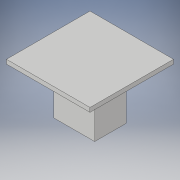
# Autodesk Inventor part: Beacon-Support
Saved by Autodesk Inventor 2017.3 (Build 213256000, 256)
## iProperties
Part Number: Beacon-Support
Material: Generisch
Document SubType Name: Modeling
Designer: Nils
Density: 1 g/cm^3
Appearance: Vorgabe
Author: Nils
Autodesk Inventor part; units mm, degrees
ref_plane "YZ Plane" through (0, 0, 0) normal (1, 0, 0) x (0, 1, 0)
ref_plane "XZ Plane" through (0, 0, 0) normal (0, 1, 0) x (-1, 0, 0)
ref_plane "XY Plane" through (0, 0, 0) normal (0, 0, 1) x (1, 0, 0)
sketch "Skizze1" plane through (0, 0, 0) normal (0, 0, 1) x (1, 0, 0)
  line L0 (-19.5, -15) -> (19.5, -15)
  line L1 (19.5, -15) -> (19.5, 15)
  line L2 (19.5, 15) -> (-19.5, 15)
  line L3 (-19.5, 15) -> (-19.5, -15)
  line L4 (-19.5, -15) -> (19.5, 15) construction
  line L5 (19.5, -15) -> (-19.5, 15) construction
  point P0 (0, 0)
  point P1 (0, 0)
  point P2 (0, 0)
  dimension "d8" = 39
  dimension "d9" = 30
  constraints: 12 end point, 3 midpoint, 2 parallel, 1 coincident, 1 horizontal, 1 perpendicular
  measures "d8" distance of L1.end L2.end
  measures "d9" distance of L0.end L1.end
extrude "Extrusion1" add sketch "Skizze1" along normal blind 47
sketch "Skizze2" plane through (0, 0, 47) normal (0, 0, 1) x (1, 0, 0)
  line L0 (-40, -40) -> (40, -40)
  line L1 (40, -40) -> (40, 40)
  line L2 (40, 40) -> (-40, 40)
  line L3 (-40, 40) -> (-40, -40)
  point P0 (0, 0)
  point P1 (0, 40)
  point P2 (-40, 0)
  dimension "d4" = 80
  constraints: 8 end point, 2 midpoint, 2 parallel, 2 perpendicular, 1 horizontal, 1 horizontal alignment, 1 vertical alignment
  measures "d4" distance of L2.end L0.start
extrude "Extrusion2" add sketch "Skizze2" along normal blind 4
